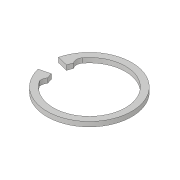
# Autodesk Inventor part: 20_Cube_Insert_Beamsplittercube_Retainring_25mm
Saved by Autodesk Inventor 2019 (Build 230136000, 136)
## iProperties
Created: 2019-08-12
Part Number: 20_Cube_Insert_Beamsplittercube_Retainring_25mm
Material: Generic
Document SubType Name: Modeling
Designer: diederichbenedict
Density: 1 g/cm^3
Appearance: Default
Author: diederichbenedict
Autodesk Inventor part; units mm, degrees
ref_plane "YZ Plane" through (0, 0, 0) normal (1, 0, 0) x (0, 1, 0)
ref_plane "XZ Plane" through (0, 0, 0) normal (0, 1, 0) x (-1, 0, 0)
ref_plane "XY Plane" through (0, 0, 0) normal (0, 0, 1) x (1, 0, 0)
sketch "Sketch1" plane through (0, 0, 0) normal (0, 1, 0) x (-1, 0, 0)
  circle A0 centre (0, 0) radius 13.5
  circle A1 centre (0, 0) radius 11.5
  line L0 (0, 0) -> (13.099, 3.2659)
  line L1 (0, 0) -> (13.099, -3.2659)
  line L2 (0, 0) -> (13.5, 0)
  circle A2 centre (0, 0) radius 10 construction
  line L3 (0, 0) -> (10.5058, 4.6775)
  line L4 (0, 0) -> (10.5058, -4.6775)
  arc A3 (9.703, 2.4192) -> (9.1355, 4.0674) centre (0, 0) ccw
  arc A4 (9.1355, -4.0674) -> (9.703, -2.4192) centre (0, 0) ccw
  arc A5 (9.1355, 4.0674) -> (9.6593, 6.2409) centre (6.4382, 5.8673) ccw
  arc A6 (9.1462, -6.9711) -> (9.1355, -4.0674) centre (7.2505, -5.5263) ccw
  circle A7 centre (11.3253, 3.4202) radius 0.5578
  circle A8 centre (11.3253, -3.4202) radius 0.5578
  point P0 (11.1584, 2.7821)
  point P1 (11.1584, -2.7821)
  dimension "d0" = 27
  dimension "d1" = 23
  dimension "d2" = 14
  dimension "d3" = 14
  dimension "d4" = 20
  dimension "d5" = 10
  dimension "d6" = 10
  constraints: 21 point on circle, 10 end point, 9 centre point, 6 point on line, 3 coincident, 2 concentric, 1 horizontal, 1 symmetric about line, 1 tangent, 1 other
  measures "d0" diameter of A0
  measures "d1" diameter of A1
  measures "d2" angle of L2 L0
  measures "d3" angle of L2 L1
  measures "d4" diameter of A2
  measures "d5" angle of L3 L0
  measures "d6" angle of L4 L1
extrude "Extrusion1" add sketch "Sketch1" along normal blind 1.5 contours L0 A1 A7 A8 L1 A0 | L0 A3 L3 A1 A7 | A1 A8 L4 A4 L1 | A7 A1 | A1 A7 | A8 A1 | A1 A8 | A5 A1 L3 | L4 A1 A6
body "Solid1"
